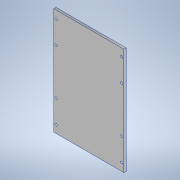
# Autodesk Inventor part: 関節2_上板
Saved by Autodesk Inventor 2021 (Build 250183000, 183)
## iProperties
Created: 2022-02-02
Part Number: 関節2_上板
Material: アルミニウム 6061
Document SubType Name: Modeling
Designer: hirohumi
Density: 2.7 g/cm^3
Appearance: アルミニウム - フラット
Mass: 126.487 g
Surface Area: 329.846 cm^2
Volume: 46.847 cm^3
Author: hirohumi
Autodesk Inventor part; units mm, degrees
ref_plane "YZ Plane" through (0, 0, 0) normal (1, 0, 0) x (0, 1, 0)
ref_plane "XZ Plane" through (0, 0, 0) normal (0, 1, 0) x (-1, 0, 0)
ref_plane "XY Plane" through (0, 0, 0) normal (0, 0, 1) x (1, 0, 0)
sketch "スケッチ1" plane through (0, 0, 0) normal (0, 0, 1) x (1, 0, 0)
  line L0 (46, 70) -> (-46, 70)
  line L1 (-46, 70) -> (-46, -70)
  line L2 (-46, -70) -> (46, -70)
  line L3 (46, -70) -> (46, 70)
  line L4 (46, 70) -> (-46, -70) construction
  line L5 (-46, 70) -> (46, -70) construction
  circle A0 centre (-43, 60) radius 1.6
  circle A1 centre (-43, 30) radius 1.6
  circle A2 centre (-43, -30) radius 1.6
  circle A3 centre (-43, -60) radius 1.6
  circle A4 centre (43, 60) radius 1.6
  circle A5 centre (43, 30) radius 1.6
  circle A6 centre (43, -30) radius 1.6
  circle A7 centre (43, -60) radius 1.6
  point P0 (0, 0)
  dimension "d0" = 92
  dimension "d1" = 140
  dimension "d2" = 3.2
  dimension "d3" = 3.2
  dimension "d4" = 3.2
  dimension "d5" = 3.2
  dimension "d6" = 120
  dimension "d7" = 10
  dimension "d8" = 30
  dimension "d9" = 30
  dimension "d10" = 3.2
  dimension "d11" = 3.2
  dimension "d12" = 3.2
  dimension "d13" = 3.2
  dimension "d14" = 120
  dimension "d15" = 30
  dimension "d16" = 30
  dimension "d17" = 3
  dimension "d18" = 3
  dimension "d19" = 60
  constraints: 12 end point, 8 centre point, 6 vertical alignment, 2 midpoint, 2 parallel, 1 horizontal, 1 perpendicular
  measures "d0" distance of L2.end L1.end
  measures "d1" distance of L1.end L0.end
  measures "d2" diameter of A0
  measures "d3" diameter of A1
  measures "d4" diameter of A2
  measures "d5" diameter of A3
  measures "d6" distance of A3.centre A0.centre
  measures "d7" distance from line of L0 A0.centre
  measures "d8" distance of A1.centre A0.centre
  measures "d9" distance of A3.centre A2.centre
  measures "d10" diameter of A4
  measures "d11" diameter of A5
  measures "d12" diameter of A6
  measures "d13" diameter of A7
  measures "d14" distance of A7.centre A4.centre
  measures "d15" distance of A5.centre A4.centre
  measures "d16" distance of A7.centre A6.centre
  measures "d17" distance from line of L1 A1.centre
  measures "d18" distance from line of L3 A5.centre
  measures "d19" vertical distance of point (0, 0) A4.centre
extrude "押し出し1" add sketch "スケッチ1" along normal blind 3
